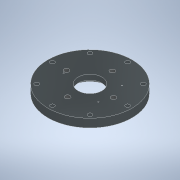
# Autodesk Inventor part: Крышка сальников
Saved by Autodesk Inventor 2021 (Build 250183000, 183)
## iProperties
Created: 2020-11-05
Part Number: Крышка сальников
Material: Чугун, серый
Document SubType Name: Modeling
Designer: Тимоха
Density: 7.15 g/cm^3
Appearance: Чугун серый
Mass: 4950.53 g
Surface Area: 904.779 cm^2
Volume: 692.382 cm^3
Author: Тимоха
Autodesk Inventor part; units mm, degrees
ref_plane "YZ Plane" through (0, 0, 0) normal (1, 0, 0) x (0, 1, 0)
ref_plane "XZ Plane" through (0, 0, 0) normal (0, 1, 0) x (-1, 0, 0)
ref_plane "XY Plane" through (0, 0, 0) normal (0, 0, 1) x (1, 0, 0)
sketch "Эскиз1" plane through (0, 0, 0) normal (0, 0, 1) x (1, 0, 0)
  line L0 (0, 30) -> (-120, 30)
  line L1 (-120, 30) -> (-120, 6)
  line L2 (-120, 6) -> (-75, 6)
  line L3 (-75, 6) -> (-75, 0)
  line L4 (-75, 0) -> (-51, 0)
  line L5 (-51, 0) -> (-51, 15)
  line L6 (-51, 15) -> (-34, 15)
  line L7 (-34, 15) -> (-34, 30)
  line L8 (0, 0) -> (0, 30)
  dimension "d31" = 120
  dimension "d32" = 24
  dimension "d33" = 45
  dimension "d34" = 24
  dimension "d35" = 15
  dimension "d36" = 17
  dimension "d38" = 30
  constraints: 18 end point, 3 perpendicular, 2 horizontal, 2 vertical, 1 point on line
  measures "d31" distance of L0.start L0.end
  measures "d32" distance of L0.end L1.end
  measures "d33" distance of L1.end L2.end
  measures "d34" distance of L3.end L4.end
  measures "d35" distance of L4.end L5.end
  measures "d36" distance of L5.end L6.end
  measures "d38" distance from line of L0 L8.start
revolve "Вращение1" add sketch "Эскиз1" angle 360 about axis through (0, 0, 0) along (0, 1, 0)
sketch "Эскиз2" plane through (0, 30, 0) normal (0, 1, 0) x (1, 0, 0)
  line L0 (0, 0) -> (0, 107.5)
  dimension "d37" = 107.5
  constraints: 2 end point, 1 vertical
  measures "d37" distance of L0.start L0.end
hole "Отверстие1" at (0, 30, -107.5) direction (0, -1, 0) diameter 12 end through all
pattern_circular "Круговой массив2" count 8 over 360 about axis through (0, 18, 0) along (0, -1, 0) of "Отверстие1"
sketch "Эскиз3" plane through (0, 30, 0) normal (0, 1, 0) x (1, 0, 0)
  line L0 (0, 0) -> (67, 0)
  circle A0 centre (67, 0) radius 2
  dimension "d39" = 67
  dimension "d40" = 4
  constraints: 2 end point, 1 centre point, 1 coincident, 1 horizontal
  measures "d39" distance of L0.start L0.end
  measures "d40" diameter of A0
extrude "Выдавливание1" cut sketch "Эскиз3" against normal through all
sketch "Эскиз4" plane through (0, 30, 0) normal (0, 1, 0) x (1, 0, 0)
  circle A0 centre (67, 0) radius 2 projected
  point P0 (0, 0)
hole "Отверстие2" at (67, 30, 0) direction (0, -1, 0) diameter 12 depth 13 tip angle 118 counterbore diameter 14 counterbore depth 11.25
thread "Резьба1" size "M14x2" class "6H" standard "ANSI Metric M Profile" full length
pattern_circular "Круговой массив3" count 2 over 360 about axis through (0, 22.5, 0) along (0, -1, 0) of "Отверстие2", "Выдавливание1"
sketch "Эскиз8" plane through (0, 30, 0) normal (0, 1, 0) x (1, 0, 0)
  line L0 (0, 0) -> (0, 64)
  circle A0 centre (0, 64) radius 4
  dimension "d66" = 64
  dimension "d67" = 8
  constraints: 2 end point, 1 centre point, 1 coincident, 1 vertical
  measures "d66" distance of L0.start L0.end
  measures "d67" diameter of A0
extrude "Выдавливание3" cut sketch "Эскиз8" against normal through all
sketch "Эскиз9" plane through (0, 30, 0) normal (0, 1, 0) x (1, 0, 0)
  circle A0 centre (0, 64) radius 4 projected
  point P0 (0, 0)
hole "Отверстие3" at (0, 30, -64) direction (0, -1, 0) diameter 12 depth 13 tip angle 118 counterbore diameter 14 counterbore depth 11.25
thread "Резьба2" size "M14x2" class "6H" standard "ANSI Metric M Profile" full length
pattern_circular "Круговой массив4" count 2 over 360 about axis through (0, 22.5, 0) along (0, -1, 0) of "Отверстие3", "Выдавливание3"
sketch "Эскиз11" plane through (0, 30, 0) normal (0, 1, 0) x (1, 0, 0)
  circle A0 centre (49.7929, 41.7812) radius 1.5 projected
  circle A1 centre (56.2917, -32.5) radius 1.5 projected
  circle A2 centre (-64.0125, -11.2871) radius 1.5 projected
  point P0 (0, 0)
extrude "Выдавливание5" cut sketch "Эскиз11" against normal blind 40
